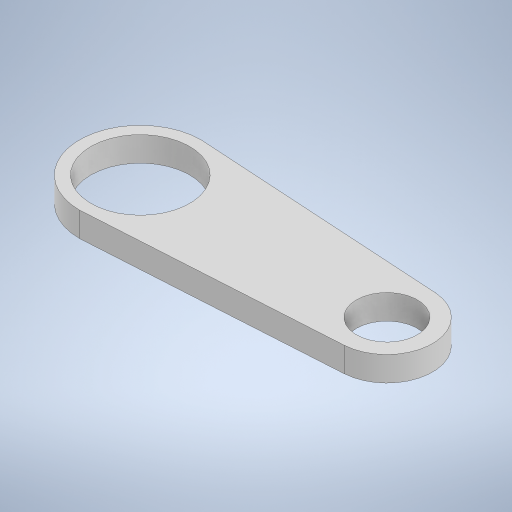
# Autodesk Inventor part: conex_llantamov
Saved by Autodesk Inventor 2024 (Build 280153000, 153)
## iProperties
Created: 2023-05-06
Part Number: conex_llantamov
Material: Generic
Document SubType Name: Modeling
Designer: Diego
Density: 1 g/cm^3
Appearance: Default
Author: Diego
Autodesk Inventor part; units mm, degrees
ref_plane "YZ Plane" through (0, 0, 0) normal (1, 0, 0) x (0, 1, 0)
ref_plane "XZ Plane" through (0, 0, 0) normal (0, 1, 0) x (-1, 0, 0)
ref_plane "XY Plane" through (0, 0, 0) normal (0, 0, 1) x (1, 0, 0)
sketch "Sketch1" plane through (0, 0, 0) normal (0, 1, 0) x (-1, 0, 0)
  circle A0 centre (0, 0) radius 6.5
  line L0 (0, 0) -> (-32.456, 0) construction
  circle A1 centre (-32.456, 0) radius 4
  arc A2 (-0.9767, -7.9402) -> (-0.9767, 7.9402) centre (0, 0) ccw
  arc A3 (-32.823, 5.9888) -> (-32.823, -5.9888) centre (-32.456, 0) ccw
  line L1 (0, 8) -> (-32.823, 5.9888)
  line L2 (0, -8) -> (-32.823, -5.9888)
  dimension "d0" = 13
  dimension "d1" = 32.456
  dimension "d2" = 8
  dimension "d3" = 16
  dimension "d4" = 12
  constraints: 6 end point, 6 point on circle, 4 centre point, 4 coincident, 2 point on line, 2 tangent, 1 horizontal
  measures "d0" diameter of A0
  measures "d1" distance of L0.start L0.end
  measures "d2" diameter of A1
  measures "d3" diameter of A2
  measures "d4" diameter of A3
extrude "Extrusion1" add sketch "Sketch1" along normal blind 3.25 contours L2 A3 L1 A2
body "Solid1"
